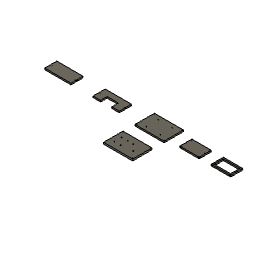
Case_modular (Autodesk Fusion 360 design; units mm, degrees)
Autodesk Fusion 360 part; units mm, degrees
sketch "Onderplaat" plane through (0, 0, 0) normal (0, 0, 1) x (1, 0, 0)
  line L0 (60, 40) -> (-60, 40)
  line L1 (-60, 40) -> (-60, -40)
  line L2 (-60, -40) -> (60, -40)
  line L3 (60, -40) -> (60, 40)
  line L4 (60, 40) -> (-60, -40) construction
  line L5 (-60, 40) -> (60, -40) construction
  dimension "d8" = 120
  dimension "d9" = 80
  constraint horizontal L0
  constraint perpendicular L0 L1
  constraint parallel L0 L2
  constraint parallel L1 L3
  constraint coincident L4 origin
  constraint coincident L5 origin
  measures "d8" distance of L1.end L2.end
  measures "d9" distance of L0.end L1.end
extrude "Extrude1" add sketch "Onderplaat" along normal blind 5.8 makes body 1
sketch "Zijkant" plane through (0, 0, 0) normal (0, 0, 1) x (1, 0, 0)
  line L0 (190, 25) -> (110, 25)
  line L1 (110, 25) -> (110, -25)
  line L2 (110, -25) -> (190, -25)
  line L3 (190, -25) -> (190, 25)
  line L4 (190, 25) -> (110, -25) construction
  line L5 (110, 25) -> (190, -25) construction
  point P0 (150, 0)
  dimension "d23" = 80
  dimension "d24" = 50
  constraint horizontal L0
  constraint perpendicular L0 L1
  constraint parallel L0 L2
  constraint parallel L1 L3
  constraint coincident L4 P0
  constraint coincident L5 P0
  measures "d23" distance of L1.end L2.end
  measures "d24" distance of L0.end L1.end
extrude "Extrude3" add sketch "Zijkant" along normal blind 5.8 separate body makes body 2
sketch "Gaten onderkant zijkant 1 " plane through (0, -25, 0) normal (0, -1, 0) x (1, 0, 0)
  line L0 (110, 0) -> (190, 0)
  line L1 (190, 0) -> (190, 5.8)
  line L2 (190, 5.8) -> (110, 5.8)
  line L3 (110, 5.8) -> (110, 0)
  line L4 (110, 5.8) -> (111.3, 5.8)
  line L5 (111.3, 5.8) -> (111.3, 4.5)
  line L6 (111.3, 4.5) -> (110, 4.5)
  line L7 (110, 4.5) -> (110, 5.8)
  line L8 (110, 0) -> (111.3, 0)
  line L9 (111.3, 0) -> (111.3, 1.3)
  line L10 (111.3, 1.3) -> (110, 1.3)
  line L11 (110, 1.3) -> (110, 0)
  line L12 (111.3, 4.5) -> (111.3, 0)
  line L13 (111.3, 4.5) -> (190, 4.5)
  line L14 (111.3, 1.3) -> (190, 1.3)
  line L15 (190, 5.8) -> (188.7, 5.8)
  line L16 (188.7, 5.8) -> (188.7, 4.5)
  line L17 (188.7, 4.5) -> (190, 4.5)
  line L18 (190, 4.5) -> (190, 5.8)
  line L19 (188.7, 4.5) -> (188.7, 0)
  line L20 (111.3, 1.3) -> (114.5, 1.3)
  line L21 (114.5, 1.3) -> (114.5, 4.5)
  circle A0 centre (112.9, 2.9) radius 1.6
  line L22 (188.7, 1.3) -> (185.5, 1.3)
  line L23 (185.5, 1.3) -> (185.5, 4.5)
  line L24 (185.5, 4.5) -> (188.7, 4.5)
  line L25 (188.7, 4.5) -> (188.7, 1.3)
  circle A1 centre (187.1, 2.9) radius 1.6
  dimension "d27" = 1.3
  dimension "d28" = 1.3
  dimension "d29" = 1.3
  dimension "d30" = 1.3
  dimension "d32" = 1.3
  dimension "d33" = 1.3
  dimension "d34" = 3.2
  dimension "d35" = 3.2
  dimension "d36" = 3.2
  dimension "d37" = 3.2
  dimension "d38" = 3.2
  constraint horizontal L4
  constraint vertical L5
  constraint horizontal L6
  constraint vertical L7
  constraint coincident L2.end L3.start
  constraint horizontal L8
  constraint vertical L9
  constraint horizontal L10
  constraint vertical L11
  constraint coincident L0.start L3.end
  constraint coincident L1 L13.end
  constraint perpendicular L1 L13
  constraint coincident L1 L14.end
  constraint perpendicular L1 L14
  constraint horizontal L15
  constraint vertical L16
  constraint horizontal L17
  constraint vertical L18
  constraint coincident L1.end L2.start
  constraint coincident L0 L19.end
  constraint perpendicular L0 L19
  constraint perpendicular L12 L20
  constraint coincident L13 L21.end
  constraint perpendicular L13 L21
  constraint horizontal L22
  constraint vertical L23
  constraint horizontal L24
  constraint vertical L25
  constraint coincident L14 L22.start
  constraint coincident L19 L22.start
  measures "d27" distance of L2.end L4.end
  measures "d28" distance of L2.end L6.end
  measures "d29" distance of L0.start L8.end
  measures "d30" distance of L0.start L10.end
  measures "d32" distance of L1.end L15.end
  measures "d33" distance of L1.end L13.end
  measures "d34" distance of L9.end L20.end
  measures "d35" diameter of A0
  measures "d36" distance of L22.start L22.end
  measures "d37" distance of L22.start L16.end
  measures "d38" diameter of A1
extrude "Extrude4" cut sketch "Gaten onderkant zijkant 1 " against normal blind 5.8 contours A0 | A1 bodies 2
sketch "Gaten bovenkant zijkant 1" plane through (0, 25, 0) normal (0, 1, 0) x (-1, 0, 0)
  line L0 (-190, 0) -> (-110, 0)
  line L1 (-110, 0) -> (-110, 5.8)
  line L2 (-110, 5.8) -> (-190, 5.8)
  line L3 (-190, 5.8) -> (-190, 0)
  line L4 (-190, 5.8) -> (-188.7, 5.8)
  line L5 (-188.7, 5.8) -> (-188.7, 4.5)
  line L6 (-188.7, 4.5) -> (-190, 4.5)
  line L7 (-190, 4.5) -> (-190, 5.8)
  line L8 (-188.7, 4.5) -> (-188.7, 0)
  line L9 (-188.7, 4.5) -> (-110, 4.5)
  line L10 (-110, 0) -> (-111.3, 0)
  line L11 (-111.3, 0) -> (-111.3, 1.3)
  line L12 (-111.3, 1.3) -> (-110, 1.3)
  line L13 (-110, 1.3) -> (-110, 0)
  line L14 (-111.3, 1.3) -> (-111.3, 4.5)
  line L15 (-111.3, 1.3) -> (-188.7, 1.3)
  line L16 (-111.3, 1.3) -> (-114.5, 1.3)
  line L17 (-114.5, 1.3) -> (-114.5, 4.5)
  line L18 (-114.5, 4.5) -> (-111.3, 4.5)
  line L19 (-111.3, 4.5) -> (-111.3, 1.3)
  line L20 (-188.7, 4.5) -> (-185.5, 4.5)
  line L21 (-185.5, 4.5) -> (-185.5, 1.3)
  line L22 (-185.5, 1.3) -> (-188.7, 1.3)
  line L23 (-188.7, 1.3) -> (-188.7, 4.5)
  circle A0 centre (-187.1, 2.9) radius 1.6
  circle A1 centre (-112.9, 2.9) radius 1.6
  dimension "d42" = 1.3
  dimension "d43" = 1.3
  dimension "d44" = 1.3
  dimension "d45" = 1.3
  dimension "d46" = 3.2
  dimension "d47" = 3.2
  dimension "d48" = 3.2
  dimension "d49" = 3.2
  dimension "d50" = 3.2
  dimension "d51" = 3.2
  constraint horizontal L4
  constraint vertical L5
  constraint horizontal L6
  constraint vertical L7
  constraint coincident L2.end L3.start
  constraint coincident L0 L8.end
  constraint perpendicular L0 L8
  constraint coincident L1 L9.end
  constraint perpendicular L1 L9
  constraint horizontal L10
  constraint vertical L11
  constraint horizontal L12
  constraint vertical L13
  constraint coincident L0.end L1.start
  constraint coincident L9 L14.end
  constraint perpendicular L9 L14
  constraint coincident L8 L15.end
  constraint perpendicular L8 L15
  constraint horizontal L16
  constraint vertical L17
  constraint horizontal L18
  constraint vertical L19
  constraint horizontal L20
  constraint vertical L21
  constraint horizontal L22
  constraint vertical L23
  measures "d42" distance of L2.end L4.end
  measures "d43" distance of L2.end L6.end
  measures "d44" distance of L0.end L10.end
  measures "d45" distance of L0.end L12.end
  measures "d46" distance of L11.end L16.end
  measures "d47" distance of L11.end L14.end
  measures "d48" distance of L5.end L20.end
  measures "d49" distance of L5.end L15.end
  measures "d50" diameter of A0
  measures "d51" diameter of A1
extrude "Extrude5" cut sketch "Gaten bovenkant zijkant 1" against normal blind 5.8 contours A0 | A1 bodies 2
sketch "Gaten onderkant" plane through (0, 0, 5.8) normal (0, 0, 1) x (-1, 0, 0)
  line L0 (-60, 40) -> (-60, -40)
  line L1 (-60, -40) -> (60, -40)
  line L2 (60, -40) -> (60, 40)
  line L3 (60, 40) -> (-60, 40)
  line L4 (-60, 40) -> (-58.7, 40)
  line L5 (-58.7, 40) -> (-58.7, 38.7)
  line L6 (-58.7, 38.7) -> (-60, 38.7)
  line L7 (-60, 38.7) -> (-60, 40)
  line L8 (-60, -40) -> (-58.7, -40)
  line L9 (-58.7, -40) -> (-58.7, -38.7)
  line L10 (-58.7, -38.7) -> (-60, -38.7)
  line L11 (-60, -38.7) -> (-60, -40)
  line L12 (-58.7, -38.7) -> (-58.7, 38.7)
  line L13 (60, 40) -> (58.7, 40)
  line L14 (58.7, 40) -> (58.7, 38.7)
  line L15 (58.7, 38.7) -> (60, 38.7)
  line L16 (60, 38.7) -> (60, 40)
  line L17 (60, -40) -> (58.7, -40)
  line L18 (58.7, -40) -> (58.7, -38.7)
  line L19 (58.7, -38.7) -> (60, -38.7)
  line L20 (60, -38.7) -> (60, -40)
  line L21 (-58.7, -38.7) -> (58.7, -38.7)
  line L22 (58.7, -38.7) -> (58.7, 38.7)
  line L23 (58.7, 38.7) -> (-58.7, 38.7)
  line L24 (-58.7, 38.7) -> (-55.5, 38.7)
  line L25 (-55.5, 38.7) -> (-55.5, 35.5)
  line L26 (-55.5, 35.5) -> (-58.7, 35.5)
  line L27 (-58.7, 35.5) -> (-58.7, 38.7)
  circle A0 centre (-57.1, 37.1) radius 1
  line L28 (58.7, 38.7) -> (55.5, 38.7)
  line L29 (55.5, 38.7) -> (55.5, 35.5)
  line L30 (55.5, 35.5) -> (58.7, 35.5)
  line L31 (58.7, 35.5) -> (58.7, 38.7)
  circle A1 centre (57.1, 37.1) radius 1
  line L32 (-58.7, -38.7) -> (-55.5, -38.7)
  line L33 (-55.5, -38.7) -> (-55.5, -35.5)
  line L34 (-55.5, -35.5) -> (-58.7, -35.5)
  line L35 (-58.7, -35.5) -> (-58.7, -38.7)
  circle A2 centre (-57.1, -37.1) radius 1
  line L36 (58.7, -38.7) -> (55.5, -38.7)
  line L37 (55.5, -38.7) -> (55.5, -35.5)
  line L38 (55.5, -35.5) -> (58.7, -35.5)
  line L39 (58.7, -35.5) -> (58.7, -38.7)
  circle A3 centre (57.1, -37.1) radius 1
  dimension "d54" = 1.3
  dimension "d55" = 1.3
  dimension "d56" = 1.3
  dimension "d57" = 1.3
  dimension "d58" = 1.3
  dimension "d59" = 1.3
  dimension "d60" = 1.3
  dimension "d61" = 1.3
  dimension "d62" = 3.2
  dimension "d63" = 3.2
  dimension "d64" = 2
  dimension "d65" = 3.2
  dimension "d66" = 3.2
  dimension "d67" = 2
  dimension "d68" = 3.2
  dimension "d69" = 3.2
  dimension "d70" = 2
  dimension "d71" = 3.2
  dimension "d72" = 3.2
  dimension "d73" = 2
  constraint horizontal L4
  constraint vertical L5
  constraint horizontal L6
  constraint vertical L7
  constraint coincident L0.start L3.end
  constraint horizontal L8
  constraint vertical L9
  constraint horizontal L10
  constraint vertical L11
  constraint coincident L0.end L1.start
  constraint horizontal L13
  constraint vertical L14
  constraint horizontal L15
  constraint vertical L16
  constraint coincident L2.end L3.start
  constraint horizontal L17
  constraint vertical L18
  constraint horizontal L19
  constraint vertical L20
  constraint coincident L1.end L2.start
  constraint horizontal L24
  constraint vertical L25
  constraint horizontal L26
  constraint vertical L27
  constraint horizontal L28
  constraint vertical L29
  constraint horizontal L30
  constraint vertical L31
  constraint horizontal L32
  constraint vertical L33
  constraint horizontal L34
  constraint vertical L35
  constraint horizontal L36
  constraint vertical L37
  constraint horizontal L38
  constraint vertical L39
  measures "d54" distance of L0.start L4.end
  measures "d55" distance of L0.start L6.end
  measures "d56" distance of L0.end L8.end
  measures "d57" distance of L0.end L10.end
  measures "d58" distance of L2.end L13.end
  measures "d59" distance of L2.end L15.end
  measures "d60" distance of L1.end L17.end
  measures "d61" distance of L1.end L19.end
  measures "d62" distance of L5.end L24.end
  measures "d63" distance of L5.end L26.end
  measures "d64" diameter of A0
  measures "d65" distance of L14.end L28.end
  measures "d66" distance of L14.end L30.end
  measures "d67" diameter of A1
  measures "d68" distance of L9.end L32.end
  measures "d69" distance of L9.end L34.end
  measures "d70" diameter of A2
  measures "d71" distance of L18.end L36.end
  measures "d72" distance of L18.end L38.end
  measures "d73" diameter of A3
extrude "Extrude6" cut sketch "Gaten onderkant" against normal blind 5.8 contours A0 | A1 | A2 | A3 bodies 1
sketch "Gaten Pi" plane through (0, 0, 5.8) normal (0, 0, 1) x (-1, 0, 0)
  circle A0 centre (57.1, 37.1) radius 1
  circle A1 centre (57.1, -37.1) radius 1
  circle A2 centre (-57.1, 37.1) radius 1
  circle A3 centre (-57.1, -37.1) radius 1
  line L0 (-60, 40) -> (-60, -40)
  line L1 (-60, -40) -> (60, -40)
  line L2 (60, -40) -> (60, 40)
  line L3 (60, 40) -> (-60, 40)
  line L4 (29, -24.5) -> (-29, 24.5) construction
  line L5 (-29, -24.5) -> (29, 24.5) construction
  circle A4 centre (-29, 24.5) radius 1.6
  circle A5 centre (29, 24.5) radius 1.6
  circle A6 centre (-29, -24.5) radius 1.6
  circle A7 centre (29, -24.5) radius 1.6
  dimension "d76" = 58
  dimension "d77" = 49
  dimension "d78" = 3.2
  dimension "d79" = 3.2
  dimension "d80" = 3.2
  dimension "d81" = 3.2
  constraint coincident L4 origin
  constraint coincident L5 origin
  constraint coincident L4.end A4.centre
  constraint coincident L5.end A5.centre
  constraint coincident L5.start A6.centre
  constraint coincident L4.start A7.centre
  measures "d76" distance of L4.end L5.end
  measures "d77" distance of L5.start L4.end
  measures "d78" diameter of A4
  measures "d79" diameter of A5
  measures "d80" diameter of A6
  measures "d81" diameter of A7
extrude "Extrude7" cut sketch "Gaten Pi" against normal blind 5.8 contours A4 | A5 | A6 | A7 bodies 1
sketch "Gaten binnenkant zijkant" plane through (0, 0, 5.8) normal (0, 0, 1) x (-1, 0, 0)
  line L0 (-190, 25) -> (-190, -25)
  line L1 (-190, -25) -> (-110, -25)
  line L2 (-110, -25) -> (-110, 25)
  line L3 (-110, 25) -> (-190, 25)
  line L4 (-190, 25) -> (-188.7, 25)
  line L5 (-188.7, 25) -> (-188.7, 23.7)
  line L6 (-188.7, 23.7) -> (-190, 23.7)
  line L7 (-190, 23.7) -> (-190, 25)
  line L8 (-190, -25) -> (-188.7, -25)
  line L9 (-188.7, -25) -> (-188.7, -23.7)
  line L10 (-188.7, -23.7) -> (-190, -23.7)
  line L11 (-190, -23.7) -> (-190, -25)
  line L12 (-110, -25) -> (-111.3, -25)
  line L13 (-111.3, -25) -> (-111.3, -23.7)
  line L14 (-111.3, -23.7) -> (-110, -23.7)
  line L15 (-110, -23.7) -> (-110, -25)
  line L16 (-110, 25) -> (-111.3, 25)
  line L17 (-111.3, 25) -> (-111.3, 23.7)
  line L18 (-111.3, 23.7) -> (-110, 23.7)
  line L19 (-110, 23.7) -> (-110, 25)
  line L20 (-188.7, 23.7) -> (-111.3, 23.7)
  line L21 (-111.3, 23.7) -> (-111.3, -23.7)
  line L22 (-111.3, -23.7) -> (-188.7, -23.7)
  line L23 (-188.7, -23.7) -> (-188.7, 23.7)
  line L24 (-111.3, 23.7) -> (-114.5, 23.7)
  line L25 (-111.3, 20.5) -> (-111.3, 23.7)
  line L26 (-111.3, -23.7) -> (-114.5, -23.7)
  line L27 (-111.3, -20.5) -> (-111.3, -23.7)
  line L28 (-188.7, 23.7) -> (-185.5, 23.7)
  line L29 (-188.7, 20.5) -> (-188.7, 23.7)
  line L30 (-188.7, -23.7) -> (-185.5, -23.7)
  line L31 (-188.7, -20.5) -> (-188.7, -23.7)
  line L32 (-185.5, -1.6) -> (-188.7, -1.6)
  line L33 (-188.7, -1.6) -> (-188.7, 1.6)
  line L34 (-188.7, 1.6) -> (-185.5, 1.6)
  line L35 (-185.5, 1.6) -> (-185.5, -1.6)
  line L36 (-185.5, -1.6) -> (-188.7, 1.6) construction
  line L37 (-188.7, -1.6) -> (-185.5, 1.6) construction
  circle A0 centre (-187.1, 0) radius 1
  line L38 (-111.3, -1.6) -> (-114.5, -1.6)
  line L39 (-114.5, -1.6) -> (-114.5, 1.6)
  line L40 (-114.5, 1.6) -> (-111.3, 1.6)
  line L41 (-111.3, 1.6) -> (-111.3, -1.6)
  line L42 (-111.3, -1.6) -> (-114.5, 1.6) construction
  line L43 (-114.5, -1.6) -> (-111.3, 1.6) construction
  circle A1 centre (-112.9, 0) radius 1
  point P0 (-187.1, 0)
  point P1 (-112.9, 0)
  dimension "d84" = 1.3
  dimension "d85" = 1.3
  dimension "d86" = 1.3
  dimension "d87" = 1.3
  dimension "d88" = 1.3
  dimension "d89" = 1.3
  dimension "d90" = 1.3
  dimension "d91" = 1.3
  dimension "d134" = 3.2
  dimension "d135" = 3.2
  dimension "d136" = 2
  dimension "d137" = 3.2
  dimension "d138" = 3.2
  dimension "d139" = 2
  constraint horizontal L4
  constraint vertical L5
  constraint horizontal L6
  constraint vertical L7
  constraint coincident L0.start L3.end
  constraint horizontal L8
  constraint vertical L9
  constraint horizontal L10
  constraint vertical L11
  constraint coincident L0.end L1.start
  constraint horizontal L12
  constraint vertical L13
  constraint horizontal L14
  constraint vertical L15
  constraint coincident L1.end L2.start
  constraint horizontal L16
  constraint vertical L17
  constraint horizontal L18
  constraint vertical L19
  constraint coincident L2.end L3.start
  constraint horizontal L24
  constraint vertical L25
  constraint horizontal L26
  constraint vertical L27
  constraint horizontal L28
  constraint vertical L29
  constraint horizontal L30
  constraint vertical L31
  constraint horizontal L32
  constraint perpendicular L32 L33
  constraint parallel L32 L34
  constraint parallel L33 L35
  constraint coincident L36 P0
  constraint coincident L37 P0
  constraint coincident P0 A0.centre
  constraint horizontal L38
  constraint perpendicular L38 L39
  constraint parallel L38 L40
  constraint parallel L39 L41
  constraint coincident L42 P1
  constraint coincident L43 P1
  constraint coincident P1 A1.centre
  measures "d84" distance of L0.start L4.end
  measures "d85" distance of L0.start L6.end
  measures "d86" distance of L0.end L8.end
  measures "d87" distance of L0.end L10.end
  measures "d88" distance of L1.end L12.end
  measures "d89" distance of L1.end L14.end
  measures "d90" distance of L2.end L16.end
  measures "d91" distance of L2.end L18.end
  measures "d134" distance of L33.end L34.end
  measures "d135" distance of L32.end L33.end
  measures "d136" diameter of A0
  measures "d137" distance of L39.end L40.end
  measures "d138" distance of L38.end L39.end
  measures "d139" diameter of A1
sketch "Voorkant" plane through (0, 0, 0) normal (0, 0, 1) x (1, 0, 0)
  line L0 (-248.4, 25) -> (-140, 25)
  line L1 (-140, 25) -> (-140, -25)
  line L2 (-140, -25) -> (-248.4, -25)
  line L3 (-248.4, -25) -> (-248.4, 25)
  line L4 (-248.4, 25) -> (-140, -25) construction
  line L5 (-140, 25) -> (-248.4, -25) construction
  point P0 (-194.2, 0)
  dimension "d104" = 108.4
  dimension "d105" = 50
  constraint horizontal L0
  constraint perpendicular L0 L1
  constraint parallel L0 L2
  constraint parallel L1 L3
  constraint coincident L4 P0
  constraint coincident L5 P0
  measures "d104" distance of L1.end L2.end
  measures "d105" distance of L0.end L1.end
extrude "Extrude8" add sketch "Voorkant" along normal blind 5.8 separate body makes body 3
sketch "Gat rechterzijkant" plane through (-140, 0, 0) normal (1, 0, 0) x (0, 1, 0)
  line L0 (-25, 0) -> (25, 0)
  line L1 (25, 0) -> (25, 5.8)
  line L2 (25, 5.8) -> (-25, 5.8)
  line L3 (-25, 5.8) -> (-25, 0)
  line L4 (-25, 5.8) -> (-23.7, 5.8)
  line L5 (-23.7, 5.8) -> (-23.7, 4.5)
  line L6 (-23.7, 4.5) -> (-25, 4.5)
  line L7 (-25, 4.5) -> (-25, 5.8)
  line L8 (-25, 0) -> (-23.7, 0)
  line L9 (-23.7, 0) -> (-23.7, 1.3)
  line L10 (-23.7, 1.3) -> (-25, 1.3)
  line L11 (-25, 1.3) -> (-25, 0)
  line L12 (25, 5.8) -> (23.7, 5.8)
  line L13 (23.7, 5.8) -> (23.7, 4.5)
  line L14 (23.7, 4.5) -> (25, 4.5)
  line L15 (25, 4.5) -> (25, 5.8)
  line L16 (25, 0) -> (23.7, 0)
  line L17 (23.7, 0) -> (23.7, 1.3)
  line L18 (23.7, 1.3) -> (25, 1.3)
  line L19 (25, 1.3) -> (25, 0)
  line L20 (-23.7, 4.5) -> (23.7, 4.5)
  line L21 (23.7, 4.5) -> (23.7, 1.3)
  line L22 (23.7, 1.3) -> (-23.7, 1.3)
  line L23 (-23.7, 1.3) -> (-23.7, 4.5)
  line L24 (1.6, 1.3) -> (-1.6, 1.3)
  line L25 (-1.6, 1.3) -> (-1.6, 4.5)
  line L26 (-1.6, 4.5) -> (1.6, 4.5)
  line L27 (1.6, 4.5) -> (1.6, 1.3)
  line L28 (1.6, 1.3) -> (-1.6, 4.5) construction
  line L29 (-1.6, 1.3) -> (1.6, 4.5) construction
  circle A0 centre (0, 2.9) radius 1.6
  point P0 (0, 2.9)
  dimension "d108" = 1.3
  dimension "d109" = 1.3
  dimension "d110" = 1.3
  dimension "d111" = 1.3
  dimension "d112" = 1.3
  dimension "d113" = 1.3
  dimension "d114" = 1.3
  dimension "d115" = 1.3
  dimension "d116" = 3.2
  dimension "d117" = 3.2
  dimension "d118" = 3.2
  constraint horizontal L4
  constraint vertical L5
  constraint horizontal L6
  constraint vertical L7
  constraint coincident L2.end L3.start
  constraint horizontal L8
  constraint vertical L9
  constraint horizontal L10
  constraint vertical L11
  constraint coincident L0.start L3.end
  constraint horizontal L12
  constraint vertical L13
  constraint horizontal L14
  constraint vertical L15
  constraint coincident L1.end L2.start
  constraint horizontal L16
  constraint vertical L17
  constraint horizontal L18
  constraint vertical L19
  constraint coincident L0.end L1.start
  constraint horizontal L24
  constraint perpendicular L24 L25
  constraint parallel L24 L26
  constraint parallel L25 L27
  constraint coincident L28 P0
  constraint coincident L29 P0
  constraint coincident P0 A0.centre
  measures "d108" distance of L2.end L4.end
  measures "d109" distance of L2.end L6.end
  measures "d110" distance of L0.start L8.end
  measures "d111" distance of L0.start L10.end
  measures "d112" distance of L1.end L12.end
  measures "d113" distance of L1.end L14.end
  measures "d114" distance of L0.end L16.end
  measures "d115" distance of L0.end L18.end
  measures "d116" distance of L25.end L26.end
  measures "d117" distance of L24.end L25.end
  measures "d118" diameter of A0
extrude "Extrude9" cut sketch "Gat rechterzijkant" against normal blind 5.8 contours A0 bodies 3
sketch "Gat linkerzijkant" plane through (-248.4, 0, 0) normal (-1, 0, 0) x (0, -1, 0)
  line L0 (-25, 0) -> (25, 0)
  line L1 (25, 0) -> (25, 5.8)
  line L2 (25, 5.8) -> (-25, 5.8)
  line L3 (-25, 5.8) -> (-25, 0)
  line L4 (-25, 5.8) -> (-23.7, 5.8)
  line L5 (-23.7, 5.8) -> (-23.7, 4.5)
  line L6 (-23.7, 4.5) -> (-25, 4.5)
  line L7 (-25, 4.5) -> (-25, 5.8)
  line L8 (-25, 0) -> (-23.7, 0)
  line L9 (-23.7, 0) -> (-23.7, 1.3)
  line L10 (-23.7, 1.3) -> (-25, 1.3)
  line L11 (-25, 1.3) -> (-25, 0)
  line L12 (25, 5.8) -> (23.7, 5.8)
  line L13 (23.7, 5.8) -> (23.7, 4.5)
  line L14 (23.7, 4.5) -> (25, 4.5)
  line L15 (25, 4.5) -> (25, 5.8)
  line L16 (25, 0) -> (23.7, 0)
  line L17 (23.7, 0) -> (23.7, 1.3)
  line L18 (23.7, 1.3) -> (25, 1.3)
  line L19 (25, 1.3) -> (25, 0)
  line L20 (-23.7, 4.5) -> (-23.7, 1.3)
  line L21 (-23.7, 1.3) -> (23.7, 1.3)
  line L22 (23.7, 1.3) -> (23.7, 4.5)
  line L23 (23.7, 4.5) -> (-23.7, 4.5)
  line L24 (1.6, 4.5) -> (-1.6, 4.5)
  line L25 (-1.6, 4.5) -> (-1.6, 1.3)
  line L26 (-1.6, 1.3) -> (1.6, 1.3)
  line L27 (1.6, 1.3) -> (1.6, 4.5)
  line L28 (1.6, 4.5) -> (-1.6, 1.3) construction
  line L29 (-1.6, 4.5) -> (1.6, 1.3) construction
  circle A0 centre (0, 2.9) radius 1.6
  point P0 (0, 2.9)
  dimension "d121" = 1.3
  dimension "d122" = 1.3
  dimension "d123" = 1.3
  dimension "d124" = 1.3
  dimension "d125" = 1.3
  dimension "d126" = 1.3
  dimension "d127" = 1.3
  dimension "d128" = 1.3
  dimension "d129" = 3.2
  dimension "d130" = 3.2
  dimension "d131" = 3.2
  constraint horizontal L4
  constraint vertical L5
  constraint horizontal L6
  constraint vertical L7
  constraint coincident L2.end L3.start
  constraint horizontal L8
  constraint vertical L9
  constraint horizontal L10
  constraint vertical L11
  constraint coincident L0.start L3.end
  constraint horizontal L12
  constraint vertical L13
  constraint horizontal L14
  constraint vertical L15
  constraint coincident L1.end L2.start
  constraint horizontal L16
  constraint vertical L17
  constraint horizontal L18
  constraint vertical L19
  constraint coincident L0.end L1.start
  constraint horizontal L24
  constraint perpendicular L24 L25
  constraint parallel L24 L26
  constraint parallel L25 L27
  constraint coincident L28 P0
  constraint coincident L29 P0
  constraint coincident P0 A0.centre
  measures "d121" distance of L2.end L4.end
  measures "d122" distance of L2.end L6.end
  measures "d123" distance of L0.start L8.end
  measures "d124" distance of L0.start L10.end
  measures "d125" distance of L1.end L12.end
  measures "d126" distance of L1.end L14.end
  measures "d127" distance of L0.end L16.end
  measures "d128" distance of L0.end L18.end
  measures "d129" distance of L25.end L26.end
  measures "d130" distance of L24.end L25.end
  measures "d131" diameter of A0
extrude "Extrude10" cut sketch "Gat linkerzijkant" against normal blind 5.8 contours A0 bodies 3
extrude "Extrude11" cut sketch "Gaten binnenkant zijkant" against normal blind 5.8 contours A0 | A1 bodies 2
copy_body "CopyPasteBodies1" bodies 3 makes body 4
move_body "Move1" bodies 4 to x (1, 0, 0) y (0, 1, 0) z (0, 0, 1) at (-200, 0, 0)
copy_body "CopyPasteBodies2" bodies 2 makes body 5
move_body "Move2" bodies 5 to x (1, 0, 0) y (0, 1, 0) z (0, 0, 1) at (130, 0, 0)
sketch "Gat usb_eth" plane through (0, 0, 5.8) normal (0, 0, 1) x (-1, 0, 0)
  circle A0 centre (-317.1, 0) radius 1
  circle A1 centre (-242.9, 0) radius 1
  line L0 (-320, 25) -> (-320, -25)
  line L1 (-320, -25) -> (-240, -25)
  line L2 (-240, -25) -> (-240, 25)
  line L3 (-240, 25) -> (-320, 25)
  line L4 (-314, 19) -> (-246, 19)
  line L5 (-246, 19) -> (-246, -19)
  line L6 (-246, -19) -> (-314, -19)
  line L7 (-314, -19) -> (-314, 19)
  line L8 (-314, 19) -> (-246, -19) construction
  line L9 (-246, 19) -> (-314, -19) construction
  point P0 (-280, 0)
  constraint horizontal L4
  constraint perpendicular L4 L5
  constraint parallel L4 L6
  constraint parallel L5 L7
  constraint coincident L8 P0
  constraint coincident L9 P0
extrude "Extrude12" cut sketch "Gat usb_eth" against normal blind 5.8 contours L4 L5 L6 L7 bodies 5
sketch "Gat GPIO" plane through (0, 0, 5.8) normal (0, 0, 1) x (-1, 0, 0)
  line L0 (248.4, 25) -> (140, 25)
  line L1 (140, 25) -> (140, -25)
  line L2 (140, -25) -> (248.4, -25)
  line L3 (248.4, -25) -> (248.4, 25)
  line L4 (212.4, 25) -> (217.4, 25)
  line L5 (217.4, 25) -> (217.4, -2)
  line L6 (176, 25.0372) -> (171, 25.0372)
  line L7 (217.4, 25) -> (171, 25.0372)
  line L8 (171, 25.0372) -> (171, -1.9628)
  line L9 (217.4, -2) -> (171, -1.9628)
  dimension "d153" = 5
  dimension "d154" = 27
  dimension "d155" = 5
  dimension "d156" = 27
  constraint perpendicular L0 L5
  measures "d153" distance of L4.start L4.end
  measures "d154" distance of L4.end L5.end
  measures "d155" distance of L6.start L6.end
  measures "d156" distance of L6.end L8.end
extrude "Extrude13" cut sketch "Gat GPIO" against normal blind 5.8 contours L0 L4 L5 L8 L9 bodies 3
sketch "Bovenplaat" plane through (0, 0, 0) normal (0, 0, 1) x (1, 0, 0)
  line L0 (60, -170) -> (-60, -170)
  line L1 (-60, -170) -> (-60, -90)
  line L2 (-60, -90) -> (60, -90)
  line L3 (60, -90) -> (60, -170)
  line L4 (60, -170) -> (-60, -90) construction
  line L5 (-60, -170) -> (60, -90) construction
  point P0 (0, -130)
  dimension "d159" = 120
  dimension "d160" = 80
  constraint horizontal L0
  constraint perpendicular L0 L1
  constraint parallel L0 L2
  constraint parallel L1 L3
  constraint coincident L4 P0
  constraint coincident L5 P0
  measures "d159" distance of L1.end L2.end
  measures "d160" distance of L0.end L1.end
extrude "Extrude14" add sketch "Bovenplaat" along normal blind 5.8 separate body makes body 6
sketch "Gaten bovenplaat" plane through (0, 0, 5.8) normal (0, 0, 1) x (-1, 0, 0)
  line L0 (-60, 90) -> (60, 90)
  line L1 (60, 90) -> (60, 170)
  line L2 (60, 170) -> (-60, 170)
  line L3 (-60, 170) -> (-60, 90)
  line L4 (60, 90) -> (58.7, 90)
  line L5 (58.7, 90) -> (58.7, 91.3)
  line L6 (58.7, 91.3) -> (60, 91.3)
  line L7 (60, 91.3) -> (60, 90)
  line L8 (60, 170) -> (58.7, 170)
  line L9 (58.7, 170) -> (58.7, 168.7)
  line L10 (58.7, 168.7) -> (60, 168.7)
  line L11 (60, 168.7) -> (60, 170)
  line L12 (-60, 170) -> (-58.7, 170)
  line L13 (-58.7, 170) -> (-58.7, 168.7)
  line L14 (-58.7, 168.7) -> (-60, 168.7)
  line L15 (-60, 168.7) -> (-60, 170)
  line L16 (-60, 90) -> (-58.7, 90)
  line L17 (-58.7, 90) -> (-58.7, 91.3)
  line L18 (-58.7, 91.3) -> (-60, 91.3)
  line L19 (-60, 91.3) -> (-60, 90)
  line L20 (58.7, 91.3) -> (-58.7, 91.3)
  line L21 (-58.7, 91.3) -> (-58.7, 168.7)
  line L22 (-58.7, 168.7) -> (58.7, 168.7)
  line L23 (58.7, 168.7) -> (58.7, 91.3)
  line L24 (58.7, 91.3) -> (55.5, 91.3)
  line L25 (55.5, 91.3) -> (55.5, 94.5)
  line L26 (55.5, 94.5) -> (58.7, 94.5)
  line L27 (58.7, 94.5) -> (58.7, 91.3)
  line L28 (-58.7, 91.3) -> (-55.5, 91.3)
  line L29 (-55.5, 91.3) -> (-55.5, 94.5)
  line L30 (-55.5, 94.5) -> (-58.7, 94.5)
  line L31 (-58.7, 94.5) -> (-58.7, 91.3)
  line L32 (-58.7, 168.7) -> (-55.5, 168.7)
  line L33 (-55.5, 168.7) -> (-55.5, 165.5)
  line L34 (-55.5, 165.5) -> (-58.7, 165.5)
  line L35 (-58.7, 165.5) -> (-58.7, 168.7)
  line L36 (58.7, 168.7) -> (55.5, 168.7)
  line L37 (55.5, 168.7) -> (55.5, 165.5)
  line L38 (55.5, 165.5) -> (58.7, 165.5)
  line L39 (58.7, 165.5) -> (58.7, 168.7)
  circle A0 centre (57.1, 167.1) radius 1
  circle A1 centre (57.1, 92.9) radius 1
  circle A2 centre (-57.1, 92.9) radius 1
  circle A3 centre (-57.1, 167.1) radius 1
  dimension "d163" = 1.3
  dimension "d164" = 1.3
  dimension "d165" = 1.3
  dimension "d166" = 1.3
  dimension "d167" = 1.3
  dimension "d168" = 1.3
  dimension "d169" = 1.3
  dimension "d170" = 1.3
  dimension "d171" = 3.2
  dimension "d172" = 3.2
  dimension "d173" = 3.2
  dimension "d174" = 3.2
  dimension "d175" = 3.2
  dimension "d176" = 3.2
  dimension "d177" = 3.2
  dimension "d178" = 3.2
  dimension "d179" = 2
  dimension "d180" = 2
  dimension "d181" = 2
  dimension "d182" = 2
  constraint horizontal L4
  constraint vertical L5
  constraint horizontal L6
  constraint vertical L7
  constraint coincident L0.end L1.start
  constraint horizontal L8
  constraint vertical L9
  constraint horizontal L10
  constraint vertical L11
  constraint coincident L1.end L2.start
  constraint horizontal L12
  constraint vertical L13
  constraint horizontal L14
  constraint vertical L15
  constraint coincident L2.end L3.start
  constraint horizontal L16
  constraint vertical L17
  constraint horizontal L18
  constraint vertical L19
  constraint coincident L0.start L3.end
  constraint horizontal L24
  constraint vertical L25
  constraint horizontal L26
  constraint vertical L27
  constraint horizontal L28
  constraint vertical L29
  constraint horizontal L30
  constraint vertical L31
  constraint horizontal L32
  constraint vertical L33
  constraint horizontal L34
  constraint vertical L35
  constraint horizontal L36
  constraint vertical L37
  constraint horizontal L38
  constraint vertical L39
  measures "d163" distance of L0.end L4.end
  measures "d164" distance of L0.end L6.end
  measures "d165" distance of L1.end L8.end
  measures "d166" distance of L1.end L10.end
  measures "d167" distance of L2.end L12.end
  measures "d168" distance of L2.end L14.end
  measures "d169" distance of L0.start L16.end
  measures "d170" distance of L0.start L18.end
  measures "d171" distance of L5.end L24.end
  measures "d172" distance of L5.end L26.end
  measures "d173" distance of L17.end L28.end
  measures "d174" distance of L17.end L30.end
  measures "d175" distance of L13.end L32.end
  measures "d176" distance of L13.end L34.end
  measures "d177" distance of L9.end L36.end
  measures "d178" distance of L9.end L38.end
  measures "d179" diameter of A0
  measures "d180" diameter of A1
  measures "d181" diameter of A2
  measures "d182" diameter of A3
extrude "Extrude15" cut sketch "Gaten bovenplaat" against normal blind 5.8 contours A0 | A1 | A2 | A3 bodies 6
extrude "Extrude16" add 1 faces at (18.7529, -142.1865, 5.8) along direction (0, 0, 1) blind 1 on bodies 6 bodies 6
sketch "Gaten relay" plane through (0, 0, 6.8) normal (0, 0, 1) x (-1, 0, 0)
  circle A0 centre (-57.1, 92.9) radius 1
  circle A1 centre (-57.1, 167.1) radius 1
  circle A2 centre (57.1, 92.9) radius 1
  circle A3 centre (57.1, 167.1) radius 1
  line L0 (-60, 90) -> (60, 90)
  line L1 (60, 90) -> (60, 170)
  line L2 (60, 170) -> (-60, 170)
  line L3 (-60, 170) -> (-60, 90)
  circle A4 centre (40, 115) radius 2
  circle A5 centre (15, 115) radius 2
  circle A6 centre (40, 145) radius 2
  circle A7 centre (15, 145) radius 2
  dimension "d193" = 25
  dimension "d194" = 30
  dimension "d195" = 4
  dimension "d196" = 4
  dimension "d197" = 4
  dimension "d198" = 4
  measures "d193" distance of A4.centre A5.centre
  measures "d194" distance of A4.centre A6.centre
  measures "d195" diameter of A4
  measures "d196" diameter of A5
  measures "d197" diameter of A6
  measures "d198" diameter of A7
extrude "Extrude17" cut sketch "Gaten relay" against normal blind 5.8 contours A4 | A5 | A6 | A7 bodies 6
sketch "Gaten stepdown" plane through (0, 0, 6.8) normal (0, 0, 1) x (-1, 0, 0)
  circle A0 centre (15, 115) radius 2
  circle A1 centre (15, 145) radius 2
  circle A2 centre (40, 115) radius 2
  circle A3 centre (40, 145) radius 2
  circle A4 centre (-57.1, 92.9) radius 1
  circle A5 centre (-57.1, 167.1) radius 1
  circle A6 centre (57.1, 92.9) radius 1
  circle A7 centre (57.1, 167.1) radius 1
  line L0 (-60, 90) -> (60, 90)
  line L1 (60, 90) -> (60, 170)
  line L2 (60, 170) -> (-60, 170)
  line L3 (-60, 170) -> (-60, 90)
  line L4 (-8, 115) -> (-32.7487, 139.7487)
  line L5 (-8, 115) -> (27, 115) construction
  circle A8 centre (-8, 115) radius 2
  circle A9 centre (-32.7487, 139.7487) radius 2
  dimension "d201" = 135
  dimension "d202" = 35
  dimension "d203" = 4
  dimension "d204" = 4
  constraint horizontal L5
  constraint coincident L4.start L5.start
  constraint coincident L4.end A9.centre
  measures "d201" angle of L4 L5
  measures "d202" distance of L4.start L4.end
  measures "d203" diameter of A8
  measures "d204" diameter of A9
extrude "Extrude18" cut sketch "Gaten stepdown" against normal blind 5.8 contours A8 | A9 bodies 6
equation "lengte = 120 mm"
equation "breedte = 80 mm"
equation "hoogte = 50 mm"
equation "dikte_boven = 5.8 mm"
equation "dikte_zijkanten = 5.8 mm"
equation "diameter_gaten_onderkant_bovenkant = 2 mm"
equation "d8 = lengte"
equation "d9 = breedte"
equation "d10 = dikte_boven"
equation "lengtegatenpi = 58 mm"
equation "breedtegatenpi = 49 mm"
equation "diameter_gaten_inserts = 3.2 mm"
equation "d23 = breedte"
equation "d24 = hoogte"
equation "d25 = dikte_zijkanten"
equation "d34 = diameter_gaten_inserts"
equation "d35 = diameter_gaten_inserts"
equation "d36 = diameter_gaten_inserts"
equation "d37 = diameter_gaten_inserts"
equation "d38 = diameter_gaten_inserts"
equation "dieptegatenzijkant = 5.8 mm"
equation "d40 = -dieptegatenzijkant"
equation "d46 = diameter_gaten_inserts"
equation "d47 = diameter_gaten_inserts"
equation "d48 = diameter_gaten_inserts"
equation "d49 = diameter_gaten_inserts"
equation "d50 = diameter_gaten_inserts"
equation "d51 = diameter_gaten_inserts"
equation "d52 = -dieptegatenzijkant"
equation "d62 = diameter_gaten_inserts"
equation "d63 = diameter_gaten_inserts"
equation "d64 = diameter_gaten_onderkant_bovenkant"
equation "d65 = diameter_gaten_inserts"
equation "d66 = diameter_gaten_inserts"
equation "d67 = diameter_gaten_onderkant_bovenkant"
equation "d68 = diameter_gaten_inserts"
equation "d69 = diameter_gaten_inserts"
equation "d70 = diameter_gaten_onderkant_bovenkant"
equation "d71 = diameter_gaten_inserts"
equation "d72 = diameter_gaten_inserts"
equation "d73 = diameter_gaten_onderkant_bovenkant"
equation "d74 = -dikte_boven"
equation "d76 = lengtegatenpi"
equation "d77 = breedtegatenpi"
equation "d78 = diameter_gaten_inserts"
equation "d79 = diameter_gaten_inserts"
equation "d80 = diameter_gaten_inserts"
equation "d81 = diameter_gaten_inserts"
equation "d82 = -dieptegatenzijkant"
equation "d104 = lengte - ( dikte_zijkanten * 2 )"
equation "d105 = hoogte"
equation "d106 = dikte_zijkanten"
equation "d116 = diameter_gaten_inserts"
equation "d117 = diameter_gaten_inserts"
equation "d118 = diameter_gaten_inserts"
equation "d119 = -dieptegatenzijkant"
equation "d129 = diameter_gaten_inserts"
equation "d130 = diameter_gaten_inserts"
equation "d131 = diameter_gaten_inserts"
equation "d132 = -dieptegatenzijkant"
equation "d134 = diameter_gaten_inserts"
equation "d135 = diameter_gaten_inserts"
equation "d136 = diameter_gaten_onderkant_bovenkant"
equation "d137 = diameter_gaten_inserts"
equation "d138 = diameter_gaten_inserts"
equation "d139 = diameter_gaten_onderkant_bovenkant"
equation "d140 = -dikte_zijkanten"
equation "d144 = -dikte_zijkanten"
equation "hoogte_gpio = 17 mm"
equation "afstand_gpio_zijkant = 36 mm"
equation "d154 = hoogte_gpio + 10 mm"
equation "d156 = hoogte_gpio + 10 mm"
equation "d157 = -dikte_zijkanten"
equation "d159 = lengte"
equation "d160 = breedte"
equation "d161 = dikte_boven"
equation "d171 = diameter_gaten_inserts"
equation "d172 = diameter_gaten_inserts"
equation "d173 = diameter_gaten_inserts"
equation "d174 = diameter_gaten_inserts"
equation "d175 = diameter_gaten_inserts"
equation "d176 = diameter_gaten_inserts"
equation "d177 = diameter_gaten_inserts"
equation "d178 = diameter_gaten_inserts"
equation "d179 = diameter_gaten_onderkant_bovenkant"
equation "d180 = diameter_gaten_onderkant_bovenkant"
equation "d181 = diameter_gaten_onderkant_bovenkant"
equation "d182 = diameter_gaten_onderkant_bovenkant"
equation "d183 = -dikte_boven"
equation "stepdown_gaten = 38.2 mm"
equation "center_stepdown = 35 mm"
equation "lengtegaten_relay = 30 mm"
equation "breedtegaten_relay = 25 mm"
equation "diameter_M3_insert = 4 mm"
equation "lengte_M3_insert = 5.8 mm"
equation "d193 = breedtegaten_relay"
equation "d194 = lengtegaten_relay"
equation "d195 = diameter_M3_insert"
equation "d196 = diameter_M3_insert"
equation "d197 = diameter_M3_insert"
equation "d198 = diameter_M3_insert"
equation "d199 = -lengte_M3_insert"
equation "d202 = center_stepdown"
equation "d203 = diameter_M3_insert"
equation "d204 = diameter_M3_insert"
equation "d205 = -lengte_M3_insert"
named bodies: "Onderplaat", "Zijkant 1", "Voorkant", "Achterkant", "Zijkant 2", "Bovenplaat"
